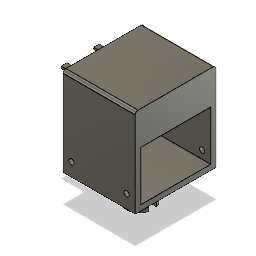
Solenoid v1 (Autodesk Fusion 360 design; units mm, degrees)
Autodesk Fusion 360 part; units mm, degrees
sketch "Sketch1" plane through (0, 0, 0) normal (0, 1, 0) x (1, 0, 0)
  line L0 (16.6624, -18.6436) -> (-16.6624, -18.6436)
  line L1 (-16.6624, -18.6436) -> (-16.6624, 18.6436)
  line L2 (-16.6624, 18.6436) -> (16.6624, 18.6436)
  line L3 (16.6624, 18.6436) -> (16.6624, -18.6436)
  line L4 (16.6624, -18.6436) -> (-16.6624, 18.6436) construction
  line L5 (-16.6624, -18.6436) -> (16.6624, 18.6436) construction
  dimension "d1" = 33.3248
  dimension "d2" = 37.2872
extrude "Extrude1" add sketch "Sketch1" along normal blind 40.8686
cylinder "CylinderPrimitive1" add diameter 12.7 height -12.7 placed x (1, 0, 0) y (0, 0, -1) z (0, 1, 0) at (0, 0, 0)
sketch "Sketch3" plane through (0, -12.7, 0) normal (0, -1, 0) x (1, 0, 0)
  circle A0 centre (0, 0) radius 6.35
  line L0 (-6.35, -1.778) -> (6.35, -1.778)
  arc A1 (6.35, -1.778) -> (6.35, 1.778) centre (6.35, 0) ccw
  line L1 (6.35, 1.778) -> (-6.35, 1.778)
  arc A2 (-6.35, 1.778) -> (-6.35, -1.778) centre (-6.35, 0) ccw
  line L2 (-6.35, 0) -> (6.35, 0) construction
extrude "Extrude2" cut sketch "Sketch3" against normal blind 9.525 contours A0 L0 L1
fillet "Fillet1" radius 1.27 2 edges at (0, 40.8686, 18.6436) (0, 40.8686, -18.6436)
hole "Hole1" at (0, -9.0033, -6.35) direction (0, 0, 1) diameter 2.4384 depth 37.2872 tip angle 180
sketch "Sketch4" plane through (0, 0, -18.6436) normal (0, 0, -1) x (-1, 0, 0)
  line L0 (16.6624, 39.5986) -> (-16.6624, 39.5986)
  line L1 (-16.6624, 39.5986) -> (-16.6624, 0)
  line L2 (-16.6624, 0) -> (16.6624, 0)
  line L3 (16.6624, 0) -> (16.6624, 39.5986)
  line L4 (0, 0) -> (0, 6.223)
  line L5 (0, 6.223) -> (12.7, 6.223)
  line L6 (12.7, 6.223) -> (0, 6.223)
  line L7 (0, 6.223) -> (-12.7, 6.223)
  dimension "d13" = 6.223
  dimension "d14" = 12.7
  measures "d13" distance of L4.start
hole "Hole2" at (12.7, 6.223, -18.6436) direction (0, 0, 1) diameter 2.4384 depth 37.2872 tip angle 180
mirror "Mirror1" about plane through (0, 0, 0) normal (1, 0, 0) of "Hole2"
sketch "Sketch5" plane through (-16.6624, 0, 0) normal (-1, 0, 0) x (0, 0, 1)
  arc A0 (-17.3736, 40.8686) -> (-18.6436, 39.5986) centre (-17.3736, 39.5986) ccw
  line L0 (-18.6436, 39.5986) -> (-18.6436, 0)
  line L1 (-18.6436, 0) -> (18.6436, 0)
  line L2 (18.6436, 0) -> (18.6436, 39.5986)
  arc A1 (18.6436, 39.5986) -> (17.3736, 40.8686) centre (17.3736, 39.5986) ccw
  line L3 (17.3736, 40.8686) -> (-17.3736, 40.8686)
  line L4 (-16.1036, 25.4052) -> (16.1036, 25.4052)
  line L5 (16.1036, 25.4052) -> (16.1036, 2.54)
  line L6 (16.1036, 2.54) -> (-16.1036, 2.54)
  line L7 (-16.1036, 2.54) -> (-16.1036, 25.4052)
  line L8 (16.1036, 13.9726) -> (18.6436, 13.9726) construction
  line L9 (-16.1036, 13.9726) -> (-18.6436, 13.9802) construction
  line L10 (0, 2.54) -> (0, 0) construction
  line L11 (0, 25.4052) -> (0, 40.8686) construction
extrude "Extrude3" cut sketch "Sketch5" against normal blind 30.8102 contours L4 L5 L6 L7
sketch "Sketch6" plane through (-16.6624, 0, 0) normal (-1, 0, 0) x (0, 0, 1)
  line L0 (16.1036, 25.4052) -> (16.1036, 2.54)
  line L1 (16.1036, 2.54) -> (-16.1036, 2.54)
  line L2 (-16.1036, 2.54) -> (-16.1036, 25.4052)
  line L3 (-16.1036, 25.4052) -> (16.1036, 25.4052)
  arc A0 (-17.3736, 40.8686) -> (-18.6436, 39.5986) centre (-17.3736, 39.5986) ccw
  line L4 (-18.6436, 39.5986) -> (-18.6436, 0)
  line L5 (-18.6436, 0) -> (18.6436, 0)
  line L6 (18.6436, 0) -> (18.6436, 39.5986)
  arc A1 (18.6436, 39.5986) -> (17.3736, 40.8686) centre (17.3736, 39.5986) ccw
  line L7 (17.3736, 40.8686) -> (-17.3736, 40.8686)
  line L8 (0, 40.8686) -> (0, 31.75) construction
  line L9 (0, 31.75) -> (7.493, 31.75) construction
  line L10 (8.89, 32.258) -> (6.096, 32.258)
  line L11 (6.096, 32.258) -> (6.096, 31.242)
  line L12 (6.096, 31.242) -> (8.89, 31.242)
  line L13 (8.89, 31.242) -> (8.89, 32.258)
  line L14 (8.89, 32.258) -> (6.096, 31.242) construction
  line L15 (6.096, 32.258) -> (8.89, 31.242) construction
  dimension "d21" = 7.493
extrude "Extrude4" add sketch "Sketch6" along normal blind 10.668 contours L10 L11 L12 L13
mirror "Mirror2" about plane through (0, 0, 0) normal (0, 0, 1) of "Extrude4"
extrude "Extrude5" cut 1 faces at (14.1478, 17.7834, 5.3679) along direction (1, 0, 0) blind 7.62
